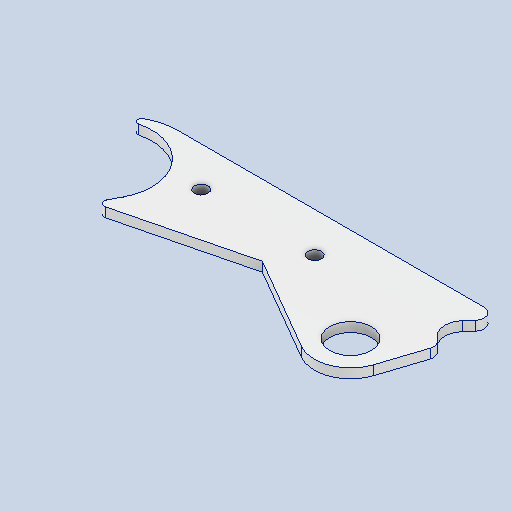
# Autodesk Inventor part: hook-bottom-plate
Saved by Autodesk Inventor 2025.2 (Build 292293000, 293)
## iProperties
Created: 2025-03-18
Part Number: hook-bottom-plate
Material: Aluminum 6061
Document SubType Name: Sheet Metal
Designer: mathe
Density: 2.7 g/cm^3
Sheet Metal Rule: Default
Appearance: Aluminum - Flat
Author: mathe
Autodesk Inventor part; units mm, degrees
ref_plane "YZ Plane" through (0, 0, 0) normal (1, 0, 0) x (0, 1, 0)
ref_plane "XZ Plane" through (0, 0, 0) normal (0, 1, 0) x (-1, 0, 0)
ref_plane "XY Plane" through (0, 0, 0) normal (0, 0, 1) x (1, 0, 0)
sketch "Sketch1" plane through (0, 0, 0) normal (0, 1, 0) x (-1, 0, 0)
  line L0 (1.8157, 35.2839) -> (-2.8584, 20.966)
  arc A0 (-2.8584, 20.966) -> (-1.9975, 17.6511) centre (0.1598, 19.9807) ccw
  line L1 (-1.9975, 17.6511) -> (-0.6941, 16.4441)
  arc A1 (-0.3495, 7.4705) -> (-0.6941, 16.4441) centre (-5.0086, 11.785) ccw
  line L2 (-0.3495, 7.4705) -> (-2.3296, 5.3323)
  arc A2 (-2.3296, 5.3323) -> (0, 0) centre (0, 3.175) ccw
  line L3 (0, 0) -> (102.7651, 0)
  arc A3 (102.7651, 0) -> (111.9831, 2.3787) centre (102.7651, 19.05) ccw
  arc A4 (111.9831, 2.3787) -> (111.0681, 4.7241) centre (111.3685, 3.4901) ccw
  arc A5 (92.5709, 28.4903) -> (111.0681, 4.7241) centre (107.1622, 20.7654) ccw
  line L4 (92.5709, 28.4903) -> (94.4719, 32.0811)
  arc A6 (94.4719, 32.0811) -> (92.6849, 34.3642) centre (93.0689, 32.8239) ccw
  line L5 (92.6849, 34.3642) -> (50.542, 23.8568)
  line L6 (50.542, 23.8568) -> (19.3436, 41.9732)
  arc A7 (19.3436, 41.9732) -> (1.8157, 35.2839) centre (13.285, 31.5396) ccw
  circle A8 centre (43.5324, 13.2882) radius 2.2479
  circle A9 centre (81.6324, 13.2882) radius 2.2479
  circle A10 centre (13.285, 31.5396) radius 6.985
  point P0 (0, 0)
  point P1 (19.3436, 41.9732)
  point P2 (-1.9975, 17.6511)
  point P3 (-0.6941, 16.4441)
  point P4 (0, 0)
  point P5 (111.9831, 2.3787)
  point P6 (111.0681, 4.7241)
extrude "Plate1" add sketch "Sketch1" along normal blind 3.175
equation "\"d0\" = Thickness"
equation "\"BendRadius\" = Thickness"
equation "\"BendReliefWidth\" = Thickness"
equation "\"BendReliefDepth\" = 0.5 * Thickness"
equation "\"CornerReliefSize\" = 4 * Thickness"
equation "\"MinimumRemnant\" = 2 * Thickness"
equation "\"TransitionRadius\" = BendRadius"
equation "\"JacobiRadiusSize\" = BendRadius"
equation "\"GapSize\" = Thickness"
equation "\"Thickness\" = 3.175"
body "Solid1"
